Autodesk Inventor part; units mm, degrees
(part 2 of 2)
sketch "Sketch26" plane through (0, 0, 0) normal (0, -1, 0) x (1, 0, 0)
  circle A0 centre (0, 0) radius 28.575 construction
  spline S0 degree 2 poles (-30.1376, 4.8959) (-29.6848, 4.8568) (-29.0206, 4.4523) (-28.8189, 4.1472) knots 0 0 0 1 2 2 2
  spline S1 degree 2 poles (-28.8189, 4.1472) (-28.5829, 3.7797) (-28.4242, 2.9776) (-28.4778, 2.3575) knots 0 0 0 1 2 2 2
  line L0 (-28.4778, 2.3575) -> (-28.6284, 0.6152)
  line L1 (-28.6284, 0.6152) -> (-34.7017, 1.1402)
  line L2 (-34.7017, 1.1402) -> (-34.5626, 2.7496)
  spline S2 degree 2 poles (-34.5626, 2.7496) (-34.5065, 3.3992) (-34.3666, 4.0417) (-34.1787, 4.3229) knots 0 0 0 1 2 2 2
  spline S3 degree 2 poles (-34.1787, 4.3229) (-33.9779, 4.6378) (-33.386, 4.8891) (-33.0021, 4.8559) knots 0 0 0 1 2 2 2
  spline S4 degree 2 poles (-33.0021, 4.8559) (-32.5739, 4.8189) (-31.9339, 4.3074) (-31.7764, 3.8921) knots 0 0 0 1 2 2 2
  line L3 (-31.7764, 3.8921) -> (-31.7468, 3.8896)
  spline S5 degree 2 poles (-31.7468, 3.8896) (-31.5524, 4.4182) (-30.7184, 4.9461) (-30.1376, 4.8959) knots 0 0 0 1 2 2 2
  spline S6 degree 2 poles (-30.1759, 4.0513) (-30.5204, 4.0811) (-30.9804, 3.9225) (-31.1634, 3.6408) knots 0 0 0 1 2 2 2
  spline S7 degree 2 poles (-31.1634, 3.6408) (-31.2784, 3.4574) (-31.3766, 3.0097) (-31.4128, 2.5914) knots 0 0 0 1 2 2 2
  line L4 (-31.4128, 2.5914) -> (-31.4919, 1.6759)
  line L5 (-31.4919, 1.6759) -> (-29.2476, 1.4819)
  line L6 (-29.2476, 1.4819) -> (-29.1911, 2.1365)
  spline S8 degree 2 poles (-29.1911, 2.1365) (-29.1451, 2.6681) (-29.1908, 3.2868) (-29.3279, 3.5367) knots 0 0 0 1 2 2 2
  spline S9 degree 2 poles (-29.3279, 3.5367) (-29.4707, 3.7771) (-29.856, 4.0237) (-30.1759, 4.0513) knots 0 0 0 1 2 2 2
  spline S10 degree 2 poles (-32.9616, 4.0045) (-33.1782, 4.0232) (-33.5158, 3.9037) (-33.6233, 3.7493) knots 0 0 0 1 2 2 2
  spline S11 degree 2 poles (-33.6233, 3.7493) (-33.7486, 3.5618) (-33.8391, 3.0887) (-33.8761, 2.6605) knots 0 0 0 1 2 2 2
  line L7 (-33.8761, 2.6605) -> (-33.9429, 1.8878)
  line L8 (-33.9429, 1.8878) -> (-32.1662, 1.7342)
  line L9 (-32.1662, 1.7342) -> (-32.0871, 2.6496)
  spline S12 degree 2 poles (-32.0871, 2.6496) (-32.0543, 3.0286) (-32.102, 3.3947) (-32.2085, 3.5973) knots 0 0 0 1 2 2 2
  spline S13 degree 2 poles (-32.2085, 3.5973) (-32.3104, 3.7945) (-32.6762, 3.9798) (-32.9616, 4.0045) knots 0 0 0 1 2 2 2
  spline S14 degree 2 poles (-29.3792, 9.6703) (-28.2597, 9.3822) (-27.3168, 7.9918) (-27.5482, 7.0924) knots 0 0 0 1 2 2 2
  spline S15 degree 2 poles (-27.5482, 7.0924) (-27.7859, 6.169) (-29.3162, 5.4356) (-30.3974, 5.7138) knots 0 0 0 1 2 2 2
  spline S16 degree 2 poles (-30.3974, 5.7138) (-31.5073, 5.9995) (-32.4561, 7.4067) (-32.2271, 8.2965) knots 0 0 0 1 2 2 2
  spline S17 degree 2 poles (-32.2271, 8.2965) (-31.9956, 9.196) (-30.4939, 9.9572) (-29.3792, 9.6703) knots 0 0 0 1 2 2 2
  spline S18 degree 2 poles (-29.5774, 8.9001) (-30.4385, 9.1217) (-31.4371, 8.7104) (-31.586, 8.1316) knots 0 0 0 1 2 2 2
  spline S19 degree 2 poles (-31.586, 8.1316) (-31.735, 7.5527) (-31.0603, 6.7057) (-30.1992, 6.4841) knots 0 0 0 1 2 2 2
  spline S20 degree 2 poles (-30.1992, 6.4841) (-29.362, 6.2686) (-28.3383, 6.6785) (-28.1893, 7.2574) knots 0 0 0 1 2 2 2
  spline S21 degree 2 poles (-28.1893, 7.2574) (-28.0416, 7.8315) (-28.7258, 8.6809) (-29.5774, 8.9001) knots 0 0 0 1 2 2 2
  spline S22 degree 2 poles (-26.2499, 11.0765) (-26.4828, 10.494) (-27.4102, 10.104) (-28.1304, 10.392) knots 0 0 0 1 2 2 2
  line L10 (-28.1304, 10.392) -> (-30.4835, 11.3329)
  line L11 (-30.4835, 11.3329) -> (-30.676, 10.8513)
  line L12 (-30.676, 10.8513) -> (-31.2678, 11.0879)
  line L13 (-31.2678, 11.0879) -> (-31.0752, 11.5695)
  line L14 (-31.0752, 11.5695) -> (-32.2953, 12.0574)
  line L15 (-32.2953, 12.0574) -> (-32.0092, 12.773)
  line L16 (-32.0092, 12.773) -> (-30.789, 12.2851)
  line L17 (-30.789, 12.2851) -> (-30.2626, 13.6015)
  line L18 (-30.2626, 13.6015) -> (-29.6709, 13.3649)
  line L19 (-29.6709, 13.3649) -> (-30.1973, 12.0485)
  line L20 (-30.1973, 12.0485) -> (-28.1745, 11.2396)
  spline S23 degree 2 poles (-28.1745, 11.2396) (-27.8534, 11.1112) (-27.4911, 10.9929) (-27.3085, 11.0104) knots 0 0 0 1 2 2 2
  spline S24 degree 2 poles (-27.3085, 11.0104) (-27.1498, 11.0214) (-26.9012, 11.2572) (-26.8022, 11.5049) knots 0 0 0 1 2 2 2
  spline S25 degree 2 poles (-26.8022, 11.5049) (-26.7325, 11.6792) (-26.7078, 12.047) (-26.7105, 12.1332) knots 0 0 0 1 2 2 2
  line L21 (-26.7105, 12.1332) -> (-26.694, 12.1745)
  line L22 (-26.694, 12.1745) -> (-26.0518, 11.9177)
  spline S26 degree 2 poles (-26.0518, 11.9177) (-26.0775, 11.6939) (-26.1784, 11.2554) (-26.2499, 11.0765) knots 0 0 0 1 2 2 2
  spline S27 degree 2 poles (-25.0386, 13.5947) (-25.3275, 13.0378) (-26.2886, 12.7405) (-26.9771, 13.0976) knots 0 0 0 1 2 2 2
  line L23 (-26.9771, 13.0976) -> (-29.2267, 14.2645)
  line L24 (-29.2267, 14.2645) -> (-29.4655, 13.8041)
  line L25 (-29.4655, 13.8041) -> (-30.0312, 14.0975)
  line L26 (-30.0312, 14.0975) -> (-29.7924, 14.558)
  line L27 (-29.7924, 14.558) -> (-30.9588, 15.163)
  line L28 (-30.9588, 15.163) -> (-30.604, 15.8471)
  line L29 (-30.604, 15.8471) -> (-29.4375, 15.2421)
  line L30 (-29.4375, 15.2421) -> (-28.7847, 16.5006)
  line L31 (-28.7847, 16.5006) -> (-28.219, 16.2072)
  line L32 (-28.219, 16.2072) -> (-28.8718, 14.9486)
  line L33 (-28.8718, 14.9486) -> (-26.938, 13.9455)
  spline S28 degree 2 poles (-26.938, 13.9455) (-26.631, 13.7863) (-26.282, 13.633) (-26.0986, 13.6325) knots 0 0 0 1 2 2 2
  spline S29 degree 2 poles (-26.0986, 13.6325) (-25.9396, 13.628) (-25.6691, 13.8383) (-25.5463, 14.0751) knots 0 0 0 1 2 2 2
  spline S30 degree 2 poles (-25.5463, 14.0751) (-25.4598, 14.2417) (-25.3992, 14.6054) (-25.3935, 14.6914) knots 0 0 0 1 2 2 2
  line L34 (-25.3935, 14.6914) -> (-25.373, 14.7309)
  line L35 (-25.373, 14.7309) -> (-24.7591, 14.4125)
  spline S31 degree 2 poles (-24.7591, 14.4125) (-24.8066, 14.1922) (-24.9499, 13.7657) (-25.0386, 13.5947) knots 0 0 0 1 2 2 2
  spline S32 degree 2 poles (-24.1836, 19.2822) (-23.2342, 18.6228) (-22.8335, 16.9913) (-23.3633, 16.2285) knots 0 0 0 1 2 2 2
  spline S33 degree 2 poles (-23.3633, 16.2285) (-23.9072, 15.4454) (-25.597, 15.2898) (-26.514, 15.9266) knots 0 0 0 1 2 2 2
  spline S34 degree 2 poles (-26.514, 15.9266) (-27.4554, 16.5803) (-27.8557, 18.2297) (-27.3316, 18.9844) knots 0 0 0 1 2 2 2
  spline S35 degree 2 poles (-27.3316, 18.9844) (-26.8018, 19.7472) (-25.129, 19.9387) (-24.1836, 19.2822) knots 0 0 0 1 2 2 2
  spline S36 degree 2 poles (-24.6373, 18.6289) (-25.3677, 19.1361) (-26.4469, 19.0977) (-26.7878, 18.6068) knots 0 0 0 1 2 2 2
  spline S37 degree 2 poles (-26.7878, 18.6068) (-27.1288, 18.1158) (-26.7907, 17.0871) (-26.0604, 16.5799) knots 0 0 0 1 2 2 2
  spline S38 degree 2 poles (-26.0604, 16.5799) (-25.3503, 16.0867) (-24.248, 16.1151) (-23.907, 16.6061) knots 0 0 0 1 2 2 2
  spline S39 degree 2 poles (-23.907, 16.6061) (-23.5689, 17.093) (-23.9151, 18.1273) (-24.6373, 18.6289) knots 0 0 0 1 2 2 2
  line L36 (-18.1124, 22.2132) -> (-19.9399, 24.1292)
  spline S40 degree 2 poles (-19.9399, 24.1292) (-20.1582, 24.358) (-20.5656, 24.7135) (-20.725, 24.7662) knots 0 0 0 1 2 2 2
  spline S41 degree 2 poles (-20.725, 24.7662) (-20.8948, 24.8296) (-21.2219, 24.736) (-21.4114, 24.5553) knots 0 0 0 1 2 2 2
  spline S42 degree 2 poles (-21.4114, 24.5553) (-21.583, 24.3916) (-21.775, 23.8057) (-21.7914, 23.4077) knots 0 0 0 1 2 2 2
  spline S43 degree 2 poles (-21.7914, 23.4077) (-21.7401, 23.3611) (-21.5999, 23.2285) (-21.5113, 23.1356) knots 0 0 0 1 2 2 2
  line L37 (-21.5113, 23.1356) -> (-19.4314, 20.955)
  line L38 (-19.4314, 20.955) -> (-19.9891, 20.4231)
  line L39 (-19.9891, 20.4231) -> (-21.8166, 22.3391)
  spline S44 degree 2 poles (-21.8166, 22.3391) (-22.0348, 22.5679) (-22.4422, 22.9235) (-22.6017, 22.9761) knots 0 0 0 1 2 2 2
  spline S45 degree 2 poles (-22.6017, 22.9761) (-22.7714, 23.0395) (-23.0986, 22.9459) (-23.2881, 22.7652) knots 0 0 0 1 2 2 2
  spline S46 degree 2 poles (-23.2881, 22.7652) (-23.4668, 22.5948) (-23.6488, 21.9911) (-23.6676, 21.6386) knots 0 0 0 1 2 2 2
  line L40 (-23.6676, 21.6386) -> (-21.3081, 19.165)
  line L41 (-21.3081, 19.165) -> (-21.8657, 18.6331)
  line L42 (-21.8657, 18.6331) -> (-25.0231, 21.9432)
  line L43 (-25.0231, 21.9432) -> (-24.4654, 22.4751)
  line L44 (-24.4654, 22.4751) -> (-24.1177, 22.1105)
  spline S47 degree 2 poles (-24.1177, 22.1105) (-24.1076, 22.5365) (-23.9071, 23.1852) (-23.6497, 23.4307) knots 0 0 0 1 2 2 2
  spline S48 degree 2 poles (-23.6497, 23.4307) (-23.3566, 23.7103) (-22.6469, 23.8752) (-22.2391, 23.6839) knots 0 0 0 1 2 2 2
  spline S49 degree 2 poles (-22.2391, 23.6839) (-22.2547, 24.2083) (-22.0518, 24.9548) (-21.773, 25.2207) knots 0 0 0 1 2 2 2
  spline S50 degree 2 poles (-21.773, 25.2207) (-21.5585, 25.4253) (-21.0821, 25.6272) (-20.8102, 25.5998) knots 0 0 0 1 2 2 2
  spline S51 degree 2 poles (-20.8102, 25.5998) (-20.5347, 25.5758) (-19.9585, 25.2652) (-19.6346, 24.9256) knots 0 0 0 1 2 2 2
  line L45 (-19.6346, 24.9256) -> (-17.5547, 22.7451)
  line L46 (-17.5547, 22.7451) -> (-18.1124, 22.2132)
  line L47 (-10.4075, 26.7042) -> (-11.1374, 26.3526)
  line L48 (-11.1374, 26.3526) -> (-12.4323, 29.0407)
  line L49 (-12.4323, 29.0407) -> (-14.9602, 27.823)
  line L50 (-14.9602, 27.823) -> (-13.6653, 25.1348)
  line L51 (-13.6653, 25.1348) -> (-14.3952, 24.7832)
  line L52 (-14.3952, 24.7832) -> (-17.0408, 30.2752)
  line L53 (-17.0408, 30.2752) -> (-16.3109, 30.6268)
  line L54 (-16.3109, 30.6268) -> (-15.2732, 28.4727)
  line L55 (-15.2732, 28.4727) -> (-12.7453, 29.6905)
  line L56 (-12.7453, 29.6905) -> (-13.783, 31.8446)
  line L57 (-13.783, 31.8446) -> (-13.0531, 32.1962)
  line L58 (-13.0531, 32.1962) -> (-10.4075, 26.7042)
  spline S52 degree 2 poles (-7.3546, 27.507) (-8.4106, 27.2112) (-9.9031, 28.0705) (-10.2096, 29.1646) knots 0 0 0 1 2 2 2
  spline S53 degree 2 poles (-10.2096, 29.1646) (-10.5108, 30.2397) (-9.7405, 31.8303) (-8.832, 32.0849) knots 0 0 0 1 2 2 2
  spline S54 degree 2 poles (-8.832, 32.0849) (-8.4229, 32.1995) (-7.7236, 32.1389) (-7.4199, 31.952) knots 0 0 0 1 2 2 2
  spline S55 degree 2 poles (-7.4199, 31.952) (-7.1114, 31.7666) (-6.6554, 31.1094) (-6.5075, 30.5814) knots 0 0 0 1 2 2 2
  line L59 (-6.5075, 30.5814) -> (-6.3942, 30.177)
  line L60 (-6.3942, 30.177) -> (-9.4433, 29.3228)
  spline S56 degree 2 poles (-9.4433, 29.3228) (-9.2288, 28.557) (-8.2303, 27.9594) (-7.5453, 28.1513) knots 0 0 0 1 2 2 2
  spline S57 degree 2 poles (-7.5453, 28.1513) (-7.3027, 28.2193) (-6.8624, 28.4606) (-6.6961, 28.5995) knots 0 0 0 1 2 2 2
  spline S58 degree 2 poles (-6.6961, 28.5995) (-6.523, 28.7507) (-6.2937, 28.9944) (-6.2247, 29.0959) knots 0 0 0 1 2 2 2
  line L61 (-6.2247, 29.0959) -> (-6.1819, 29.1079)
  line L62 (-6.1819, 29.1079) -> (-5.9553, 28.2992)
  spline S59 degree 2 poles (-5.9553, 28.2992) (-6.0691, 28.2109) (-6.4165, 27.9494) (-6.5567, 27.8639) knots 0 0 0 1 2 2 2
  spline S60 degree 2 poles (-6.5567, 27.8639) (-6.7535, 27.7421) (-7.0882, 27.5817) (-7.3546, 27.507) knots 0 0 0 1 2 2 2
  spline S61 degree 2 poles (-7.2758, 30.5405) (-7.3693, 30.8376) (-7.6156, 31.2406) (-7.7758, 31.3547) knots 0 0 0 1 2 2 2
  spline S62 degree 2 poles (-7.7758, 31.3547) (-7.9509, 31.4852) (-8.4045, 31.5479) (-8.7042, 31.464) knots 0 0 0 1 2 2 2
  spline S63 degree 2 poles (-8.7042, 31.464) (-8.9991, 31.3814) (-9.3637, 31.0894) (-9.4869, 30.8702) knots 0 0 0 1 2 2 2
  spline S64 degree 2 poles (-9.4869, 30.8702) (-9.6041, 30.6476) (-9.6568, 30.1762) (-9.6019, 29.8889) knots 0 0 0 1 2 2 2
  line L63 (-9.6019, 29.8889) -> (-7.2758, 30.5405)
  line L64 (-1.5038, 28.6079) -> (-2.4401, 28.4915)
  line L65 (-2.4401, 28.4915) -> (-3.7551, 30.0605)
  line L66 (-3.7551, 30.0605) -> (-4.6756, 28.2138)
  line L67 (-4.6756, 28.2138) -> (-5.5433, 28.106)
  line L68 (-5.5433, 28.106) -> (-4.2493, 30.5517)
  line L69 (-4.2493, 30.5517) -> (-6.0927, 32.6473)
  line L70 (-6.0927, 32.6473) -> (-5.1563, 32.7637)
  line L71 (-5.1563, 32.7637) -> (-3.8481, 31.2088)
  line L72 (-3.8481, 31.2088) -> (-2.9356, 33.0396)
  line L73 (-2.9356, 33.0396) -> (-2.0679, 33.1475)
  line L74 (-2.0679, 33.1475) -> (-3.3533, 30.7128)
  line L75 (-3.3533, 30.7128) -> (-1.5038, 28.6079)
  line L76 (0.5107, 31.9833) -> (-0.4674, 31.9839)
  line L77 (-0.4674, 31.9839) -> (-0.4667, 33.1498)
  line L78 (-0.4667, 33.1498) -> (0.5115, 33.1491)
  line L79 (0.5115, 33.1491) -> (0.5107, 31.9833)
  line L80 (0.5084, 28.5747) -> (-0.4697, 28.5753)
  line L81 (-0.4697, 28.5753) -> (-0.469, 29.7412)
  line L82 (-0.469, 29.7412) -> (0.5092, 29.7405)
  line L83 (0.5092, 29.7405) -> (0.5084, 28.5747)
  spline S65 degree 2 poles (8.9249, 30.4001) (8.5607, 28.801) (7.2899, 27.5147) (6.3217, 27.7352) knots 0 0 0 1 2 2 2
  spline S66 degree 2 poles (6.3217, 27.7352) (5.3391, 27.959) (4.7669, 29.6954) (5.1234, 31.2609) knots 0 0 0 1 2 2 2
  spline S67 degree 2 poles (5.1234, 31.2609) (5.4898, 32.8696) (6.7584, 34.1463) (7.7313, 33.9247) knots 0 0 0 1 2 2 2
  spline S68 degree 2 poles (7.7313, 33.9247) (8.7091, 33.702) (9.2781, 31.9511) (8.9249, 30.4001) knots 0 0 0 1 2 2 2
  spline S69 degree 2 poles (7.4912, 28.8216) (7.6738, 29.0891) (7.9763, 29.9727) (8.1157, 30.5844) knots 0 0 0 1 2 2 2
  spline S70 degree 2 poles (8.1157, 30.5844) (8.255, 31.1962) (8.3638, 32.1188) (8.3125, 32.4497) knots 0 0 0 1 2 2 2
  spline S71 degree 2 poles (8.3125, 32.4497) (8.2612, 32.7806) (7.9134, 33.1891) (7.5811, 33.2648) knots 0 0 0 1 2 2 2
  spline S72 degree 2 poles (7.5811, 33.2648) (7.2487, 33.3405) (6.7487, 33.125) (6.5522, 32.8405) knots 0 0 0 1 2 2 2
  spline S73 degree 2 poles (6.5522, 32.8405) (6.3627, 32.5644) (6.0653, 31.6594) (5.9326, 31.0766) knots 0 0 0 1 2 2 2
  spline S74 degree 2 poles (5.9326, 31.0766) (5.79, 30.4504) (5.6762, 29.5947) (5.7268, 29.2387) knots 0 0 0 1 2 2 2
  spline S75 degree 2 poles (5.7268, 29.2387) (5.7722, 28.9041) (6.1252, 28.4741) (6.472, 28.3951) knots 0 0 0 1 2 2 2
  spline S76 degree 2 poles (6.472, 28.3951) (6.7995, 28.3205) (7.2995, 28.536) (7.4912, 28.8216) knots 0 0 0 1 2 2 2
  line L84 (10.2051, 26.695) -> (9.2857, 27.0287)
  line L85 (9.2857, 27.0287) -> (9.6835, 28.1246)
  line L86 (9.6835, 28.1246) -> (10.6029, 27.7908)
  line L87 (10.6029, 27.7908) -> (10.2051, 26.695)
  spline S77 degree 2 poles (15.5351, 26.3257) (15.335, 25.9342) (14.7426, 25.3937) (14.3879, 25.2643) knots 0 0 0 1 2 2 2
  spline S78 degree 2 poles (14.3879, 25.2643) (14.0333, 25.1349) (13.2053, 25.1974) (12.7831, 25.4133) knots 0 0 0 1 2 2 2
  spline S79 degree 2 poles (12.7831, 25.4133) (12.396, 25.6111) (11.727, 26.1693) (11.5196, 26.4473) knots 0 0 0 1 2 2 2
  line L88 (11.5196, 26.4473) -> (11.913, 27.2171)
  line L89 (11.913, 27.2171) -> (11.9658, 27.1901)
  spline S80 degree 2 poles (11.9658, 27.1901) (12.0179, 27.0858) (12.2493, 26.7679) (12.4025, 26.6008) knots 0 0 0 1 2 2 2
  spline S81 degree 2 poles (12.4025, 26.6008) (12.5798, 26.4159) (12.8934, 26.1502) (13.1177, 26.0355) knots 0 0 0 1 2 2 2
  spline S82 degree 2 poles (13.1177, 26.0355) (13.3377, 25.9231) (13.8321, 25.8702) (14.0693, 25.9653) knots 0 0 0 1 2 2 2
  spline S83 degree 2 poles (14.0693, 25.9653) (14.2889, 26.0583) (14.65, 26.4175) (14.7984, 26.7078) knots 0 0 0 1 2 2 2
  spline S84 degree 2 poles (14.7984, 26.7078) (14.9467, 26.9981) (14.9772, 27.4486) (14.8906, 27.6482) knots 0 0 0 1 2 2 2
  spline S85 degree 2 poles (14.8906, 27.6482) (14.8063, 27.8632) (14.4073, 28.2114) (14.1302, 28.353) knots 0 0 0 1 2 2 2
  spline S86 degree 2 poles (14.1302, 28.353) (13.8311, 28.5059) (13.19, 28.717) (12.9894, 28.7696) knots 0 0 0 1 2 2 2
  line L90 (12.9894, 28.7696) -> (14.4193, 31.5673)
  line L91 (14.4193, 31.5673) -> (17.3973, 30.0453)
  line L92 (17.3973, 30.0453) -> (17.0713, 29.4074)
  line L93 (17.0713, 29.4074) -> (14.7927, 30.572)
  line L94 (14.7927, 30.572) -> (14.0531, 29.1248)
  spline S87 degree 2 poles (14.0531, 29.1248) (14.194, 29.0749) (14.4559, 28.9577) (14.5615, 28.9038) knots 0 0 0 1 2 2 2
  spline S88 degree 2 poles (14.5615, 28.9038) (14.9793, 28.6902) (15.4859, 28.2593) (15.6464, 27.9221) knots 0 0 0 1 2 2 2
  spline S89 degree 2 poles (15.6464, 27.9221) (15.8113, 27.5826) (15.7869, 26.8184) (15.5351, 26.3257) knots 0 0 0 1 2 2 2
  line L95 (18.4323, 21.9193) -> (15.3996, 24.1408)
  line L96 (15.3996, 24.1408) -> (15.9105, 24.8382)
  spline S90 degree 2 poles (15.9105, 24.8382) (16.462, 24.9057) (17.4613, 25.0494) (17.9651, 25.1519) knots 0 0 0 1 2 2 2
  spline S91 degree 2 poles (17.9651, 25.1519) (18.9795, 25.358) (19.9329, 25.7985) (20.2219, 26.1931) knots 0 0 0 1 2 2 2
  spline S92 degree 2 poles (20.2219, 26.1931) (20.3737, 26.4003) (20.4739, 26.8046) (20.4313, 26.9889) knots 0 0 0 1 2 2 2
  spline S93 degree 2 poles (20.4313, 26.9889) (20.3887, 27.1731) (20.1588, 27.4946) (19.9755, 27.6289) knots 0 0 0 1 2 2 2
  spline S94 degree 2 poles (19.9755, 27.6289) (19.8002, 27.7574) (19.3773, 27.9324) (19.1643, 27.9844) knots 0 0 0 1 2 2 2
  spline S95 degree 2 poles (19.1643, 27.9844) (18.9839, 28.0308) (18.6081, 28.0611) (18.4875, 28.0637) knots 0 0 0 1 2 2 2
  line L97 (18.4875, 28.0637) -> (18.4517, 28.09)
  line L98 (18.4517, 28.09) -> (18.9654, 28.7914)
  spline S96 degree 2 poles (18.9654, 28.7914) (19.2417, 28.7421) (20.114, 28.4032) (20.4408, 28.1638) knots 0 0 0 1 2 2 2
  spline S97 degree 2 poles (20.4408, 28.1638) (21.1302, 27.6587) (21.3731, 26.3602) (20.9177, 25.7385) knots 0 0 0 1 2 2 2
  spline S98 degree 2 poles (20.9177, 25.7385) (20.7046, 25.4476) (20.213, 25.0606) (19.9416, 24.941) knots 0 0 0 1 2 2 2
  spline S99 degree 2 poles (19.9416, 24.941) (19.6644, 24.8134) (19.0083, 24.6449) (18.6681, 24.5818) knots 0 0 0 1 2 2 2
  spline S100 degree 2 poles (18.6681, 24.5818) (18.1091, 24.4708) (16.8166, 24.303) (16.4348, 24.2582) knots 0 0 0 1 2 2 2
  line L99 (16.4348, 24.2582) -> (18.8498, 22.4891)
  line L100 (18.8498, 22.4891) -> (18.4323, 21.9193)
  line L101 (21.6843, 18.7082) -> (19.0435, 21.3839)
  line L102 (19.0435, 21.3839) -> (19.6588, 21.9911)
  spline S101 degree 2 poles (19.6588, 21.9911) (20.2141, 21.97) (21.2235, 21.9529) (21.7372, 21.974) knots 0 0 0 1 2 2 2
  spline S102 degree 2 poles (21.7372, 21.974) (22.7714, 22.0161) (23.7828, 22.2994) (24.1309, 22.6429) knots 0 0 0 1 2 2 2
  spline S103 degree 2 poles (24.1309, 22.6429) (24.3138, 22.8234) (24.477, 23.2066) (24.4642, 23.3953) knots 0 0 0 1 2 2 2
  spline S104 degree 2 poles (24.4642, 23.3953) (24.4515, 23.584) (24.2757, 23.938) (24.116, 24.0997) knots 0 0 0 1 2 2 2
  spline S105 degree 2 poles (24.116, 24.0997) (23.9634, 24.2544) (23.5737, 24.4945) (23.3717, 24.5797) knots 0 0 0 1 2 2 2
  spline S106 degree 2 poles (23.3717, 24.5797) (23.201, 24.6541) (22.8348, 24.7439) (22.7162, 24.7656) knots 0 0 0 1 2 2 2
  line L103 (22.7162, 24.7656) -> (22.6849, 24.7973)
  line L104 (22.6849, 24.7973) -> (23.3037, 25.408)
  spline S107 degree 2 poles (23.3037, 25.408) (23.5686, 25.3154) (24.3759, 24.842) (24.6605, 24.5537) knots 0 0 0 1 2 2 2
  spline S108 degree 2 poles (24.6605, 24.5537) (25.2608, 23.9455) (25.294, 22.6248) (24.7455, 22.0835) knots 0 0 0 1 2 2 2
  spline S109 degree 2 poles (24.7455, 22.0835) (24.4889, 21.8302) (23.9419, 21.5263) (23.655, 21.4514) knots 0 0 0 1 2 2 2
  spline S110 degree 2 poles (23.655, 21.4514) (23.361, 21.3695) (22.6864, 21.3075) (22.3406, 21.2993) knots 0 0 0 1 2 2 2
  spline S111 degree 2 poles (22.3406, 21.2993) (21.771, 21.2786) (20.4683, 21.3186) (20.0842, 21.3351) knots 0 0 0 1 2 2 2
  line L105 (20.0842, 21.3351) -> (22.1871, 19.2044)
  line L106 (22.1871, 19.2044) -> (21.6843, 18.7082)
  spline S112 degree 2 poles (25.9239, 16.1968) (25.5658, 15.9416) (24.7909, 15.7352) (24.4165, 15.7839) knots 0 0 0 1 2 2 2
  spline S113 degree 2 poles (24.4165, 15.7839) (24.0422, 15.8326) (23.3363, 16.2698) (23.0611, 16.6561) knots 0 0 0 1 2 2 2
  spline S114 degree 2 poles (23.0611, 16.6561) (22.8089, 17.0101) (22.4727, 17.8139) (22.4168, 18.1562) knots 0 0 0 1 2 2 2
  line L107 (22.4168, 18.1562) -> (23.1209, 18.6579)
  line L108 (23.1209, 18.6579) -> (23.1553, 18.6096)
  spline S115 degree 2 poles (23.1553, 18.6096) (23.1534, 18.493) (23.2121, 18.1042) (23.271, 17.8853) knots 0 0 0 1 2 2 2
  spline S116 degree 2 poles (23.271, 17.8853) (23.3431, 17.6395) (23.4989, 17.2591) (23.645, 17.0539) knots 0 0 0 1 2 2 2
  spline S117 degree 2 poles (23.645, 17.0539) (23.7884, 16.8528) (24.2027, 16.5778) (24.4571, 16.5528) knots 0 0 0 1 2 2 2
  spline S118 degree 2 poles (24.4571, 16.5528) (24.6948, 16.5341) (25.1808, 16.6863) (25.4463, 16.8755) knots 0 0 0 1 2 2 2
  spline S119 degree 2 poles (25.4463, 16.8755) (25.7119, 17.0647) (25.9466, 17.4504) (25.9618, 17.6674) knots 0 0 0 1 2 2 2
  spline S120 degree 2 poles (25.9618, 17.6674) (25.9862, 17.8971) (25.7926, 18.39) (25.612, 18.6435) knots 0 0 0 1 2 2 2
  spline S121 degree 2 poles (25.612, 18.6435) (25.4171, 18.9171) (24.9456, 19.4) (24.7919, 19.5392) knots 0 0 0 1 2 2 2
  line L109 (24.7919, 19.5392) -> (27.3507, 21.3623)
  line L110 (27.3507, 21.3623) -> (29.2914, 18.6386)
  line L111 (29.2914, 18.6386) -> (28.708, 18.223)
  line L112 (28.708, 18.223) -> (27.2231, 20.307)
  line L113 (27.2231, 20.307) -> (25.8994, 19.3639)
  spline S122 degree 2 poles (25.8994, 19.3639) (26.0015, 19.2546) (26.1799, 19.0299) (26.2487, 18.9333) knots 0 0 0 1 2 2 2
  spline S123 degree 2 poles (26.2487, 18.9333) (26.521, 18.5511) (26.7718, 17.9352) (26.7587, 17.562) knots 0 0 0 1 2 2 2
  spline S124 degree 2 poles (26.7587, 17.562) (26.7485, 17.1847) (26.3745, 16.5178) (25.9239, 16.1968) knots 0 0 0 1 2 2 2
  line L114 (26.8479, 9.8544) -> (25.9436, 12.0357)
  line L115 (25.9436, 12.0357) -> (26.5186, 12.2741)
  line L116 (26.5186, 12.2741) -> (26.8156, 11.5576)
  line L117 (26.8156, 11.5576) -> (31.297, 13.4153)
  line L118 (31.297, 13.4153) -> (30.9999, 14.1318)
  line L119 (30.9999, 14.1318) -> (31.5749, 14.3701)
  line L120 (31.5749, 14.3701) -> (32.4792, 12.1888)
  line L121 (32.4792, 12.1888) -> (31.9042, 11.9505)
  line L122 (31.9042, 11.9505) -> (31.6072, 12.6669)
  line L123 (31.6072, 12.6669) -> (27.1259, 10.8092)
  line L124 (27.1259, 10.8092) -> (27.4229, 10.0927)
  line L125 (27.4229, 10.0927) -> (26.8479, 9.8544)
  spline S125 degree 2 poles (31.3296, 4.9821) (30.5185, 4.7844) (29.0527, 5.1236) (28.5534, 5.5866) knots 0 0 0 1 2 2 2
  spline S126 degree 2 poles (28.5534, 5.5866) (28.1602, 5.9687) (27.7424, 6.8482) (27.5669, 7.5681) knots 0 0 0 1 2 2 2
  line L126 (27.5669, 7.5681) -> (27.2345, 8.9311)
  line L127 (27.2345, 8.9311) -> (33.157, 10.3752)
  line L128 (33.157, 10.3752) -> (33.4858, 9.0265)
  spline S127 degree 2 poles (33.4858, 9.0265) (33.6895, 8.1914) (33.6716, 7.1803) (33.5327, 6.7905) knots 0 0 0 1 2 2 2
  spline S128 degree 2 poles (33.5327, 6.7905) (33.2928, 6.1269) (32.1935, 5.1928) (31.3296, 4.9821) knots 0 0 0 1 2 2 2
  spline S129 degree 2 poles (31.1391, 5.8052) (31.8206, 5.9713) (32.6753, 6.6577) (32.84, 7.1708) knots 0 0 0 1 2 2 2
  spline S130 degree 2 poles (32.84, 7.1708) (32.95, 7.5332) (32.9436, 8.2892) (32.8137, 8.822) knots 0 0 0 1 2 2 2
  line L129 (32.8137, 8.822) -> (32.6674, 9.4219)
  line L130 (32.6674, 9.4219) -> (28.1079, 8.3102)
  line L131 (28.1079, 8.3102) -> (28.2542, 7.7103)
  spline S131 degree 2 poles (28.2542, 7.7103) (28.3818, 7.1871) (28.7428, 6.4362) (29.0468, 6.1696) knots 0 0 0 1 2 2 2
  spline S132 degree 2 poles (29.0468, 6.1696) (29.4258, 5.8247) (30.448, 5.6367) (31.1391, 5.8052) knots 0 0 0 1 2 2 2
  line L132 (28.5071, 2.0292) -> (28.4209, 3.0035)
  line L133 (28.4209, 3.0035) -> (29.5822, 3.1062)
  line L134 (29.5822, 3.1062) -> (29.6684, 2.1318)
  line L135 (29.6684, 2.1318) -> (28.5071, 2.0292)
  line L136 (31.9024, 2.3293) -> (31.8163, 3.3037)
  line L137 (31.8163, 3.3037) -> (32.9776, 3.4063)
  line L138 (32.9776, 3.4063) -> (33.0638, 2.432)
  line L139 (33.0638, 2.432) -> (31.9024, 2.3293)
  line L140 (28.0978, -5.4439) -> (28.4983, -2.4971)
  line L141 (28.4983, -2.4971) -> (29.1151, -2.5809)
  line L142 (29.1151, -2.5809) -> (28.9661, -3.6774)
  line L143 (28.9661, -3.6774) -> (33.0143, -4.2276)
  line L144 (33.0143, -4.2276) -> (33.1633, -3.1311)
  line L145 (33.1633, -3.1311) -> (33.7164, -3.2063)
  spline S133 degree 2 poles (33.7164, -3.2063) (33.6319, -3.8279) (33.9045, -4.4632) (34.3887, -4.5689) knots 0 0 0 1 2 2 2
  line L146 (34.3887, -4.5689) -> (34.3036, -5.1955)
  line L147 (34.3036, -5.1955) -> (28.8603, -4.4557)
  line L148 (28.8603, -4.4557) -> (28.7146, -5.5277)
  line L149 (28.7146, -5.5277) -> (28.0978, -5.4439)
  line L150 (27.4952, -7.7961) -> (27.746, -6.8507)
  line L151 (27.746, -6.8507) -> (28.8729, -7.1497)
  line L152 (28.8729, -7.1497) -> (28.6221, -8.0951)
  line L153 (28.6221, -8.0951) -> (27.4952, -7.7961)
  spline S134 degree 2 poles (27.6004, -13.1378) (27.1927, -12.9733) (26.6017, -12.4311) (26.4414, -12.0894) knots 0 0 0 1 2 2 2
  spline S135 degree 2 poles (26.4414, -12.0894) (26.281, -11.7476) (26.2698, -10.9174) (26.4473, -10.4776) knots 0 0 0 1 2 2 2
  spline S136 degree 2 poles (26.4473, -10.4776) (26.61, -10.0745) (27.1067, -9.3587) (27.3652, -9.1274) knots 0 0 0 1 2 2 2
  line L154 (27.3652, -9.1274) -> (28.1669, -9.451)
  line L155 (28.1669, -9.451) -> (28.1447, -9.5059)
  spline S137 degree 2 poles (28.1447, -9.5059) (28.0454, -9.5671) (27.7492, -9.8258) (27.5964, -9.9932) knots 0 0 0 1 2 2 2
  spline S138 degree 2 poles (27.5964, -9.9932) (27.4279, -10.1862) (27.1911, -10.5221) (27.0968, -10.7558) knots 0 0 0 1 2 2 2
  spline S139 degree 2 poles (27.0968, -10.7558) (27.0044, -10.9848) (26.9955, -11.482) (27.1113, -11.7098) knots 0 0 0 1 2 2 2
  spline S140 degree 2 poles (27.1113, -11.7098) (27.2235, -11.9203) (27.6132, -12.2481) (27.9156, -12.3701) knots 0 0 0 1 2 2 2
  spline S141 degree 2 poles (27.9156, -12.3701) (28.2179, -12.4921) (28.6693, -12.4825) (28.8604, -12.3785) knots 0 0 0 1 2 2 2
  spline S142 degree 2 poles (28.8604, -12.3785) (29.0671, -12.2755) (29.3785, -11.8472) (29.495, -11.5586) knots 0 0 0 1 2 2 2
  spline S143 degree 2 poles (29.495, -11.5586) (29.6208, -11.2471) (29.7742, -10.5898) (29.8087, -10.3854) knots 0 0 0 1 2 2 2
  line L156 (29.8087, -10.3854) -> (32.7222, -11.5613)
  line L157 (32.7222, -11.5613) -> (31.4705, -14.6626)
  line L158 (31.4705, -14.6626) -> (30.8062, -14.3945)
  line L159 (30.8062, -14.3945) -> (31.764, -12.0216)
  line L160 (31.764, -12.0216) -> (30.2569, -11.4133)
  spline S144 degree 2 poles (30.2569, -11.4133) (30.2197, -11.5581) (30.1262, -11.8293) (30.0819, -11.9393) knots 0 0 0 1 2 2 2
  spline S145 degree 2 poles (30.0819, -11.9393) (29.9062, -12.3745) (29.522, -12.9173) (29.2003, -13.1071) knots 0 0 0 1 2 2 2
  spline S146 degree 2 poles (29.2003, -13.1071) (28.8768, -13.3014) (28.1134, -13.3449) (27.6004, -13.1378) knots 0 0 0 1 2 2 2
  line L161 (29.6765, -18.4873) -> (27.7102, -17.1502)
  line L162 (27.7102, -17.1502) -> (27.9788, -16.6835)
  line L163 (27.9788, -16.6835) -> (30.1226, -17.7123)
  line L164 (30.1226, -17.7123) -> (29.6765, -18.4873)
  line L165 (30.4454, -17.1515) -> (28.4791, -15.8144)
  line L166 (28.4791, -15.8144) -> (28.7477, -15.3477)
  line L167 (28.7477, -15.3477) -> (30.8915, -16.3765)
  line L168 (30.8915, -16.3765) -> (30.4454, -17.1515)
  spline S147 degree 2 poles (22.8704, -25.2005) (22.3391, -25.1635) (21.223, -24.608) (20.6801, -24.0751) knots 0 0 0 1 2 2 2
  spline S148 degree 2 poles (20.6801, -24.0751) (20.1513, -23.556) (19.5576, -22.4472) (19.5177, -21.9096) knots 0 0 0 1 2 2 2
  spline S149 degree 2 poles (19.5177, -21.9096) (19.4775, -21.344) (19.8839, -20.3517) (20.3027, -19.9251) knots 0 0 0 1 2 2 2
  spline S150 degree 2 poles (20.3027, -19.9251) (20.7352, -19.4844) (21.727, -19.0734) (22.2722, -19.1033) knots 0 0 0 1 2 2 2
  spline S151 degree 2 poles (22.2722, -19.1033) (22.807, -19.1368) (23.9196, -19.7028) (24.4555, -20.2288) knots 0 0 0 1 2 2 2
  spline S152 degree 2 poles (24.4555, -20.2288) (25.0019, -20.7652) (25.5675, -21.8533) (25.6215, -22.3978) knots 0 0 0 1 2 2 2
  spline S153 degree 2 poles (25.6215, -22.3978) (25.6614, -22.9354) (25.2655, -23.9381) (24.8364, -24.3753) knots 0 0 0 1 2 2 2
  spline S154 degree 2 poles (24.8364, -24.3753) (24.4004, -24.8195) (23.3911, -25.2271) (22.8704, -25.2005) knots 0 0 0 1 2 2 2
  spline S155 degree 2 poles (21.2718, -23.4722) (21.702, -23.8944) (22.5517, -24.3616) (22.9364, -24.4069) knots 0 0 0 1 2 2 2
  spline S156 degree 2 poles (22.9364, -24.4069) (23.3315, -24.4556) (24.0347, -24.1906) (24.3323, -23.8874) knots 0 0 0 1 2 2 2
  spline S157 degree 2 poles (24.3323, -23.8874) (24.6403, -23.5736) (24.8854, -22.8867) (24.8292, -22.4785) knots 0 0 0 1 2 2 2
  spline S158 degree 2 poles (24.8292, -22.4785) (24.7767, -22.0877) (24.2868, -21.2469) (23.8638, -20.8317) knots 0 0 0 1 2 2 2
  spline S159 degree 2 poles (23.8638, -20.8317) (23.0071, -19.9908) (21.3916, -19.8171) (20.7998, -20.42) knots 0 0 0 1 2 2 2
  spline S160 degree 2 poles (20.7998, -20.42) (20.2081, -21.0228) (20.4152, -22.6313) (21.2718, -23.4722) knots 0 0 0 1 2 2 2
  spline S161 degree 2 poles (15.5041, -27.6765) (15.0381, -26.9837) (14.8498, -25.4911) (15.1117, -24.8625) knots 0 0 0 1 2 2 2
  spline S162 degree 2 poles (15.1117, -24.8625) (15.3343, -24.3615) (16.0152, -23.6654) (16.6301, -23.2518) knots 0 0 0 1 2 2 2
  line L169 (16.6301, -23.2518) -> (17.7942, -22.4689)
  line L170 (17.7942, -22.4689) -> (21.1964, -27.5272)
  line L171 (21.1964, -27.5272) -> (20.0445, -28.3019)
  spline S163 degree 2 poles (20.0445, -28.3019) (19.3313, -28.7816) (18.3763, -29.1143) (17.9625, -29.1188) knots 0 0 0 1 2 2 2
  spline S164 degree 2 poles (17.9625, -29.1188) (17.2569, -29.123) (16.0003, -28.4143) (15.5041, -27.6765) knots 0 0 0 1 2 2 2
  spline S165 degree 2 poles (16.2105, -27.2132) (16.602, -27.7953) (17.5415, -28.3601) (18.0799, -28.3373) knots 0 0 0 1 2 2 2
  spline S166 degree 2 poles (18.0799, -28.3373) (18.4579, -28.3152) (19.1652, -28.0479) (19.6202, -27.7419) knots 0 0 0 1 2 2 2
  line L172 (19.6202, -27.7419) -> (20.1326, -27.3973)
  line L173 (20.1326, -27.3973) -> (17.5134, -23.5031)
  line L174 (17.5134, -23.5031) -> (17.0011, -23.8477)
  spline S167 degree 2 poles (17.0011, -23.8477) (16.5543, -24.1482) (15.9744, -24.7466) (15.8293, -25.124) knots 0 0 0 1 2 2 2
  spline S168 degree 2 poles (15.8293, -25.124) (15.6367, -25.5988) (15.8135, -26.623) (16.2105, -27.2132) knots 0 0 0 1 2 2 2
  line L175 (13.2128, -29.131) -> (14.0973, -28.7134)
  line L176 (14.0973, -28.7134) -> (14.595, -29.7676)
  line L177 (14.595, -29.7676) -> (13.7105, -30.1852)
  line L178 (13.7105, -30.1852) -> (13.2128, -29.131)
  line L179 (11.7575, -26.0486) -> (12.642, -25.631)
  line L180 (12.642, -25.631) -> (13.1398, -26.6853)
  line L181 (13.1398, -26.6853) -> (12.2553, -27.1029)
  line L182 (12.2553, -27.1029) -> (11.7575, -26.0486)
  spline S169 degree 2 poles (7.5616, -33.2445) (7.7786, -33.1964) (8.1844, -32.9953) (8.3736, -32.8674) knots 0 0 0 1 2 2 2
  spline S170 degree 2 poles (8.3736, -32.8674) (8.5484, -32.7427) (8.7945, -32.5061) (8.8884, -32.4043) knots 0 0 0 1 2 2 2
  line L183 (8.8884, -32.4043) -> (8.9366, -32.3937)
  line L184 (8.9366, -32.3937) -> (9.1235, -33.2377)
  spline S171 degree 2 poles (9.1235, -33.2377) (8.894, -33.4353) (8.0519, -33.8595) (7.6515, -33.9481) knots 0 0 0 1 2 2 2
  spline S172 degree 2 poles (7.6515, -33.9481) (7.2464, -34.0378) (6.6072, -34.0073) (6.3227, -33.8881) knots 0 0 0 1 2 2 2
  spline S173 degree 2 poles (6.3227, -33.8881) (6.0206, -33.7576) (5.6299, -33.2724) (5.5487, -32.9058) knots 0 0 0 1 2 2 2
  spline S174 degree 2 poles (5.5487, -32.9058) (5.4398, -32.4138) (5.9217, -31.528) (6.3538, -31.3311) knots 0 0 0 1 2 2 2
  line L185 (6.3538, -31.3311) -> (6.341, -31.2733)
  spline S175 degree 2 poles (6.341, -31.2733) (6.1443, -31.2763) (5.6766, -31.1977) (5.4549, -31.0646) knots 0 0 0 1 2 2 2
  spline S176 degree 2 poles (5.4549, -31.0646) (5.2342, -30.9364) (4.8831, -30.4474) (4.7966, -30.0568) knots 0 0 0 1 2 2 2
  spline S177 degree 2 poles (4.7966, -30.0568) (4.708, -29.6564) (4.8324, -28.9155) (5.0256, -28.5995) knots 0 0 0 1 2 2 2
  spline S178 degree 2 poles (5.0256, -28.5995) (5.2262, -28.2718) (5.9023, -27.8286) (6.3701, -27.7251) knots 0 0 0 1 2 2 2
  spline S179 degree 2 poles (6.3701, -27.7251) (6.8187, -27.6258) (7.7446, -27.6485) (8.0767, -27.7318) knots 0 0 0 1 2 2 2
  line L186 (8.0767, -27.7318) -> (8.2635, -28.5759)
  line L187 (8.2635, -28.5759) -> (8.2057, -28.5887)
  spline S180 degree 2 poles (8.2057, -28.5887) (7.9143, -28.461) (6.9906, -28.3112) (6.571, -28.4041) knots 0 0 0 1 2 2 2
  spline S181 degree 2 poles (6.571, -28.4041) (6.325, -28.4586) (5.8672, -28.7218) (5.7427, -28.9366) knots 0 0 0 1 2 2 2
  spline S182 degree 2 poles (5.7427, -28.9366) (5.6231, -29.1503) (5.5482, -29.6121) (5.6198, -29.9353) knots 0 0 0 1 2 2 2
  spline S183 degree 2 poles (5.6198, -29.9353) (5.6913, -30.2584) (5.9723, -30.6364) (6.1678, -30.7196) knots 0 0 0 1 2 2 2
  spline S184 degree 2 poles (6.1678, -30.7196) (6.3633, -30.8028) (6.8418, -30.793) (7.1119, -30.7333) knots 0 0 0 1 2 2 2
  line L188 (7.1119, -30.7333) -> (7.4495, -30.6585)
  line L189 (7.4495, -30.6585) -> (7.5958, -31.3193)
  line L190 (7.5958, -31.3193) -> (7.3305, -31.378)
  spline S185 degree 2 poles (7.3305, -31.378) (6.7951, -31.4965) (6.2331, -32.1573) (6.3409, -32.6444) knots 0 0 0 1 2 2 2
  spline S186 degree 2 poles (6.3409, -32.6444) (6.3911, -32.8711) (6.6363, -33.1559) (6.7975, -33.2214) knots 0 0 0 1 2 2 2
  spline S187 degree 2 poles (6.7975, -33.2214) (6.9694, -33.2895) (7.3542, -33.2904) (7.5616, -33.2445) knots 0 0 0 1 2 2 2
  line L191 (2.1881, -28.4952) -> (3.1619, -28.4038)
  line L192 (3.1619, -28.4038) -> (3.2709, -29.5646)
  line L193 (3.2709, -29.5646) -> (2.297, -29.656)
  line L194 (2.297, -29.656) -> (2.1881, -28.4952)
  line L195 (-2.7928, -28.5027) -> (0.9648, -28.6181)
  line L196 (0.9648, -28.6181) -> (0.9382, -29.4822)
  spline S188 degree 2 poles (0.9382, -29.4822) (0.5217, -29.85) (-0.2209, -30.5339) (-0.5782, -30.9035) knots 0 0 0 1 2 2 2
  spline S189 degree 2 poles (-0.5782, -30.9035) (-1.2979, -31.6475) (-1.8347, -32.5503) (-1.8497, -33.0391) knots 0 0 0 1 2 2 2
  spline S190 degree 2 poles (-1.8497, -33.0391) (-1.8576, -33.2959) (-1.7114, -33.6859) (-1.572, -33.8137) knots 0 0 0 1 2 2 2
  spline S191 degree 2 poles (-1.572, -33.8137) (-1.4326, -33.9415) (-1.0612, -34.0765) (-0.834, -34.0835) knots 0 0 0 1 2 2 2
  spline S192 degree 2 poles (-0.834, -34.0835) (-0.6168, -34.0901) (-0.169, -33.9952) (0.036, -33.9174) knots 0 0 0 1 2 2 2
  spline S193 degree 2 poles (0.036, -33.9174) (0.2109, -33.8536) (0.538, -33.666) (0.6388, -33.5999) knots 0 0 0 1 2 2 2
  line L197 (0.6388, -33.5999) -> (0.6833, -33.6012)
  line L198 (0.6833, -33.6012) -> (0.6566, -34.4703)
  spline S194 degree 2 poles (0.6566, -34.4703) (0.401, -34.586) (-0.5101, -34.8002) (-0.915, -34.7877) knots 0 0 0 1 2 2 2
  spline S195 degree 2 poles (-0.915, -34.7877) (-1.7692, -34.7615) (-2.7043, -33.8284) (-2.6806, -33.0581) knots 0 0 0 1 2 2 2
  spline S196 degree 2 poles (-2.6806, -33.0581) (-2.6696, -32.6976) (-2.4832, -32.1004) (-2.3272, -31.8482) knots 0 0 0 1 2 2 2
  spline S197 degree 2 poles (-2.3272, -31.8482) (-2.1708, -31.5861) (-1.7252, -31.0759) (-1.4805, -30.8313) knots 0 0 0 1 2 2 2
  spline S198 degree 2 poles (-1.4805, -30.8313) (-1.0824, -30.4234) (-0.1117, -29.5537) (0.1778, -29.3007) knots 0 0 0 1 2 2 2
  line L199 (0.1778, -29.3007) -> (-2.8145, -29.2088)
  line L200 (-2.8145, -29.2088) -> (-2.7928, -28.5027)
  spline S199 degree 2 poles (-7.5946, -29.6092) (-7.5114, -29.1775) (-7.0928, -28.4935) (-6.7882, -28.2705) knots 0 0 0 1 2 2 2
  spline S200 degree 2 poles (-6.7882, -28.2705) (-6.4836, -28.0475) (-5.6709, -27.8771) (-5.2052, -27.9669) knots 0 0 0 1 2 2 2
  spline S201 degree 2 poles (-5.2052, -27.9669) (-4.7784, -28.0492) (-3.9805, -28.3992) (-3.7039, -28.6085) knots 0 0 0 1 2 2 2
  line L201 (-3.7039, -28.6085) -> (-3.8676, -29.4573)
  line L202 (-3.8676, -29.4573) -> (-3.9258, -29.4461)
  spline S202 degree 2 poles (-3.9258, -29.4461) (-4.0048, -29.3604) (-4.3156, -29.1194) (-4.5092, -29.0016) knots 0 0 0 1 2 2 2
  spline S203 degree 2 poles (-4.5092, -29.0016) (-4.731, -28.8733) (-5.1061, -28.7054) (-5.3535, -28.6577) knots 0 0 0 1 2 2 2
  spline S204 degree 2 poles (-5.3535, -28.6577) (-5.596, -28.611) (-6.0857, -28.6977) (-6.2871, -28.8551) knots 0 0 0 1 2 2 2
  spline S205 degree 2 poles (-6.2871, -28.8551) (-6.472, -29.0056) (-6.7189, -29.451) (-6.7806, -29.7712) knots 0 0 0 1 2 2 2
  spline S206 degree 2 poles (-6.7806, -29.7712) (-6.8423, -30.0913) (-6.7463, -30.5324) (-6.6075, -30.7) knots 0 0 0 1 2 2 2
  spline S207 degree 2 poles (-6.6075, -30.7) (-6.4667, -30.8831) (-5.9866, -31.1065) (-5.681, -31.1654) knots 0 0 0 1 2 2 2
  spline S208 degree 2 poles (-5.681, -31.1654) (-5.3511, -31.229) (-4.6766, -31.2534) (-4.4694, -31.2481) knots 0 0 0 1 2 2 2
  line L203 (-4.4694, -31.2481) -> (-5.0641, -34.3331)
  line L204 (-5.0641, -34.3331) -> (-8.348, -33.7001)
  line L205 (-8.348, -33.7001) -> (-8.2124, -32.9967)
  line L206 (-8.2124, -32.9967) -> (-5.6998, -33.4811)
  line L207 (-5.6998, -33.4811) -> (-5.3921, -31.8852)
  spline S209 degree 2 poles (-5.3921, -31.8852) (-5.5414, -31.8766) (-5.8255, -31.8369) (-5.9419, -31.8144) knots 0 0 0 1 2 2 2
  spline S210 degree 2 poles (-5.9419, -31.8144) (-6.4027, -31.7256) (-7.0092, -31.4527) (-7.2572, -31.1735) knots 0 0 0 1 2 2 2
  spline S211 degree 2 poles (-7.2572, -31.1735) (-7.5101, -30.8933) (-7.6993, -30.1525) (-7.5946, -29.6092) knots 0 0 0 1 2 2 2
  line L208 (-12.4459, -32.6737) -> (-11.5113, -30.4873)
  line L209 (-11.5113, -30.4873) -> (-11.0017, -30.6613)
  line L210 (-11.0017, -30.6613) -> (-11.5998, -32.9627)
  line L211 (-11.5998, -32.9627) -> (-12.4459, -32.6737)
  line L212 (-10.9874, -33.1719) -> (-10.0527, -30.9854)
  line L213 (-10.0527, -30.9854) -> (-9.5431, -31.1595)
  line L214 (-9.5431, -31.1595) -> (-10.1412, -33.4609)
  line L215 (-10.1412, -33.4609) -> (-10.9874, -33.1719)
  line L216 (-17.4703, -22.7204) -> (-16.7919, -23.1632)
  line L217 (-16.7919, -23.1632) -> (-18.4226, -25.6619)
  line L218 (-18.4226, -25.6619) -> (-16.0728, -27.1954)
  line L219 (-16.0728, -27.1954) -> (-14.4421, -24.6967)
  line L220 (-14.4421, -24.6967) -> (-13.7636, -25.1395)
  line L221 (-13.7636, -25.1395) -> (-17.0952, -30.2445)
  line L222 (-17.0952, -30.2445) -> (-17.7737, -29.8017)
  line L223 (-17.7737, -29.8017) -> (-16.4669, -27.7994)
  line L224 (-16.4669, -27.7994) -> (-18.8168, -26.2659)
  line L225 (-18.8168, -26.2659) -> (-20.1235, -28.2682)
  line L226 (-20.1235, -28.2682) -> (-20.802, -27.8254)
  line L227 (-20.802, -27.8254) -> (-17.4703, -22.7204)
  spline S212 degree 2 poles (-19.3142, -20.9453) (-18.8451, -21.3618) (-18.7923, -22.3665) (-19.3072, -22.9465) knots 0 0 0 1 2 2 2
  line L228 (-19.3072, -22.9465) -> (-20.9897, -24.8417)
  line L229 (-20.9897, -24.8417) -> (-20.6018, -25.1861)
  line L230 (-20.6018, -25.1861) -> (-21.0248, -25.6626)
  line L231 (-21.0248, -25.6626) -> (-21.4127, -25.3183)
  line L232 (-21.4127, -25.3183) -> (-22.2851, -26.3009)
  line L233 (-22.2851, -26.3009) -> (-22.8614, -25.7893)
  line L234 (-22.8614, -25.7893) -> (-21.9891, -24.8066)
  line L235 (-21.9891, -24.8066) -> (-23.0493, -23.8654)
  line L236 (-23.0493, -23.8654) -> (-22.6263, -23.3888)
  line L237 (-22.6263, -23.3888) -> (-21.566, -24.3301)
  line L238 (-21.566, -24.3301) -> (-20.1197, -22.7009)
  spline S213 degree 2 poles (-20.1197, -22.7009) (-19.8901, -22.4423) (-19.656, -22.1414) (-19.6106, -21.9637) knots 0 0 0 1 2 2 2
  spline S214 degree 2 poles (-19.6106, -21.9637) (-19.5672, -21.8107) (-19.7049, -21.4969) (-19.9044, -21.3198) knots 0 0 0 1 2 2 2
  spline S215 degree 2 poles (-19.9044, -21.3198) (-20.0447, -21.1952) (-20.3825, -21.0473) (-20.4645, -21.0207) knots 0 0 0 1 2 2 2
  line L239 (-20.4645, -21.0207) -> (-20.4978, -20.9912)
  line L240 (-20.4978, -20.9912) -> (-20.0386, -20.474)
  spline S216 degree 2 poles (-20.0386, -20.474) (-19.8367, -20.574) (-19.4583, -20.8174) (-19.3142, -20.9453) knots 0 0 0 1 2 2 2
  line L241 (-21.3573, -18.9904) -> (-20.695, -19.7101)
  line L242 (-20.695, -19.7101) -> (-21.5528, -20.4996)
  line L243 (-21.5528, -20.4996) -> (-22.2152, -19.7799)
  line L244 (-22.2152, -19.7799) -> (-21.3573, -18.9904)
  line L245 (-23.8655, -21.2986) -> (-23.2031, -22.0183)
  line L246 (-23.2031, -22.0183) -> (-24.061, -22.8078)
  line L247 (-24.061, -22.8078) -> (-24.7233, -22.0881)
  line L248 (-24.7233, -22.0881) -> (-23.8655, -21.2986)
  spline S217 degree 2 poles (-29.4771, -17.1312) (-29.3665, -17.324) (-29.0535, -17.6513) (-28.875, -17.7938) knots 0 0 0 1 2 2 2
  spline S218 degree 2 poles (-28.875, -17.7938) (-28.7038, -17.9235) (-28.4045, -18.0878) (-28.2794, -18.1471) knots 0 0 0 1 2 2 2
  line L249 (-28.2794, -18.1471) -> (-28.2549, -18.1899)
  line L250 (-28.2549, -18.1899) -> (-29.0048, -18.62)
  spline S219 degree 2 poles (-29.0048, -18.62) (-29.2618, -18.4598) (-29.9178, -17.7825) (-30.1218, -17.4269) knots 0 0 0 1 2 2 2
  spline S220 degree 2 poles (-30.1218, -17.4269) (-30.3282, -17.0669) (-30.4897, -16.4476) (-30.4608, -16.1406) knots 0 0 0 1 2 2 2
  spline S221 degree 2 poles (-30.4608, -16.1406) (-30.4263, -15.8134) (-30.0797, -15.2957) (-29.754, -15.1089) knots 0 0 0 1 2 2 2
  spline S222 degree 2 poles (-29.754, -15.1089) (-29.3169, -14.8583) (-28.3276, -15.0541) (-28.0109, -15.4078) knots 0 0 0 1 2 2 2
  line L251 (-28.0109, -15.4078) -> (-27.9595, -15.3783)
  spline S223 degree 2 poles (-27.9595, -15.3783) (-28.0211, -15.1915) (-28.0855, -14.7216) (-28.0246, -14.4703) knots 0 0 0 1 2 2 2
  spline S224 degree 2 poles (-28.0246, -14.4703) (-27.968, -14.2214) (-27.606, -13.7405) (-27.2589, -13.5414) knots 0 0 0 1 2 2 2
  spline S225 degree 2 poles (-27.2589, -13.5414) (-26.9032, -13.3375) (-26.1589, -13.2352) (-25.7997, -13.3254) knots 0 0 0 1 2 2 2
  spline S226 degree 2 poles (-25.7997, -13.3254) (-25.427, -13.4192) (-24.8024, -13.9323) (-24.5641, -14.348) knots 0 0 0 1 2 2 2
  spline S227 degree 2 poles (-24.5641, -14.348) (-24.3355, -14.7466) (-24.0811, -15.6371) (-24.0616, -15.979) knots 0 0 0 1 2 2 2
  line L252 (-24.0616, -15.979) -> (-24.8115, -16.409)
  line L253 (-24.8115, -16.409) -> (-24.841, -16.3576)
  spline S228 degree 2 poles (-24.841, -16.3576) (-24.806, -16.0414) (-24.9385, -15.1151) (-25.1523, -14.7423) knots 0 0 0 1 2 2 2
  spline S229 degree 2 poles (-25.1523, -14.7423) (-25.2776, -14.5237) (-25.6654, -14.1652) (-25.9075, -14.1105) knots 0 0 0 1 2 2 2
  spline S230 degree 2 poles (-25.9075, -14.1105) (-26.1472, -14.06) (-26.6103, -14.1262) (-26.8974, -14.2909) knots 0 0 0 1 2 2 2
  spline S231 degree 2 poles (-26.8974, -14.2909) (-27.1846, -14.4555) (-27.4616, -14.8365) (-27.4827, -15.0479) knots 0 0 0 1 2 2 2
  spline S232 degree 2 poles (-27.4827, -15.0479) (-27.5038, -15.2593) (-27.3518, -15.7131) (-27.2142, -15.9531) knots 0 0 0 1 2 2 2
  line L254 (-27.2142, -15.9531) -> (-27.0421, -16.2531)
  line L255 (-27.0421, -16.2531) -> (-27.6292, -16.5898)
  line L256 (-27.6292, -16.5898) -> (-27.7644, -16.3541)
  spline S233 degree 2 poles (-27.7644, -16.3541) (-28.0372, -15.8784) (-28.8355, -15.5389) (-29.2683, -15.7871) knots 0 0 0 1 2 2 2
  spline S234 degree 2 poles (-29.2683, -15.7871) (-29.4697, -15.9026) (-29.6684, -16.2215) (-29.6828, -16.395) knots 0 0 0 1 2 2 2
  spline S235 degree 2 poles (-29.6828, -16.395) (-29.6966, -16.5794) (-29.5827, -16.9469) (-29.4771, -17.1312) knots 0 0 0 1 2 2 2
  line L257 (-26.5462, -10.5859) -> (-26.1686, -11.4882)
  line L258 (-26.1686, -11.4882) -> (-27.2441, -11.9383)
  line L259 (-27.2441, -11.9383) -> (-27.6217, -11.036)
  line L260 (-27.6217, -11.036) -> (-26.5462, -10.5859)
  spline S236 degree 2 poles (-30.9839, -6.6198) (-29.4041, -6.179) (-27.6681, -6.6844) (-27.4012, -7.6408) knots 0 0 0 1 2 2 2
  spline S237 degree 2 poles (-27.4012, -7.6408) (-27.1303, -8.6115) (-28.3851, -9.9412) (-29.9315, -10.3727) knots 0 0 0 1 2 2 2
  spline S238 degree 2 poles (-29.9315, -10.3727) (-31.5208, -10.8162) (-33.2474, -10.3081) (-33.5156, -9.3469) knots 0 0 0 1 2 2 2
  spline S239 degree 2 poles (-33.5156, -9.3469) (-33.7851, -8.381) (-32.516, -7.0473) (-30.9839, -6.6198) knots 0 0 0 1 2 2 2
  spline S240 degree 2 poles (-28.9133, -7.1293) (-29.2354, -7.0961) (-30.1565, -7.2505) (-30.7608, -7.4192) knots 0 0 0 1 2 2 2
  spline S241 degree 2 poles (-30.7608, -7.4192) (-31.3651, -7.5878) (-32.2284, -7.9312) (-32.4949, -8.1338) knots 0 0 0 1 2 2 2
  spline S242 degree 2 poles (-32.4949, -8.1338) (-32.7615, -8.3364) (-32.9553, -8.8367) (-32.8637, -9.165) knots 0 0 0 1 2 2 2
  spline S243 degree 2 poles (-32.8637, -9.165) (-32.7721, -9.4933) (-32.3446, -9.8305) (-32.0008, -9.8679) knots 0 0 0 1 2 2 2
  spline S244 degree 2 poles (-32.0008, -9.8679) (-31.6678, -9.9033) (-30.7303, -9.734) (-30.1546, -9.5733) knots 0 0 0 1 2 2 2
  spline S245 degree 2 poles (-30.1546, -9.5733) (-29.536, -9.4007) (-28.7293, -9.0936) (-28.4403, -8.8796) knots 0 0 0 1 2 2 2
  spline S246 degree 2 poles (-28.4403, -8.8796) (-28.1676, -8.6804) (-27.9575, -8.1653) (-28.0531, -7.8227) knots 0 0 0 1 2 2 2
  spline S247 degree 2 poles (-28.0531, -7.8227) (-28.1434, -7.4991) (-28.5708, -7.1619) (-28.9133, -7.1293) knots 0 0 0 1 2 2 2
  line L261 (-34.589, -4.9698) -> (-32.2152, -4.8305)
  line L262 (-32.2152, -4.8305) -> (-32.1436, -5.3642)
  line L263 (-32.1436, -5.3642) -> (-34.47, -5.856)
  line L264 (-34.47, -5.856) -> (-34.589, -4.9698)
  line L265 (-34.7941, -3.4422) -> (-32.4203, -3.303)
  line L266 (-32.4203, -3.303) -> (-32.3486, -3.8366)
  line L267 (-32.3486, -3.8366) -> (-34.6751, -4.3284)
  line L268 (-34.6751, -4.3284) -> (-34.7941, -3.4422)
  dimension "d145" = 57.15
  constraints: 1 centre point, 1 coincident, 1 other
  measures "d145" diameter of A0
extrude "Extrusion19" cut sketch "Sketch26" against normal blind 1.27
split "Split1" plane through (0, 38.1, 0) removes the side toward (0, -1, 0)
equation "\"d85\" = spoolExteriorRadius"
equation "\"d86\" = spoolOverallHeight"
equation "\"d88\" = d85"
equation "\"d89\" = 0.5 * spoolOverallHeight"
equation "\"centerLineForSpool\" = 0.25 * spoolOverallHeight"
equation "\"d103\" = hexDiameter"
equation "\"d110\" = centerLineForSpool"
equation "\"d111\" = centerLineForSpool"
equation "\"d112\" = holeForString"
equation "\"d121\" = centerLineForSpool"
equation "\"d122\" = holeForString"
equation "\"d125\" = knotHoleDiameter"
equation "\"d127\" = holeForString"
equation "\"d128\" = centerLineForSpool"
equation "\"d129\" = knotHoleDiameter"
equation "\"d130\" = knotHoleDepth"
equation "\"d132\" = hexHoleChamfer"
equation "\"holeForString\" = stringDiameter + clearanceForString"
equation "\"stringDiameter\" = 3.048"
equation "\"clearanceForString\" = 2.032"
equation "\"spoolHeightWithoutSpacer\" = 69.85"
equation "\"hexShaftDiameter\" = 12.7"
equation "\"clearanceForHexShaft\" = 0.5715"
equation "\"hexDiameter\" = hexShaftDiameter + clearanceForHexShaft"
equation "\"supportChannels\" = 3.81"
equation "\"spoolInteriorDiameter\" = 38.1"
equation "\"spoolInteriroRadius\" = 0.5 * spoolInteriorDiameter"
equation "\"spoolExteriorDiameter\" = 82.55"
equation "\"spoolExteriorRadius\" = 0.5 * spoolExteriorDiameter"
equation "\"spoolFiletRadius\" = 0.5 * supportChannels"
equation "\"holeCenter\" = 0.25 * spoolHeightWithoutSpacer - 0.75 * supportChannels"
equation "\"hexHoleChamfer\" = 1.5875"
equation "\"stringHoleCenterFromHexShaft\" = 0.5 * hexDiameter + 0.5 * holeForString"
equation "\"textCircleDiameter\" = 0.75 * spoolExteriorDiameter"
equation "\"textHeight\" = 6.096"
equation "\"textDepth\" = 1.27"
equation "\"stringHoleChamfer\" = 4.7625"
equation "\"spoolTotalHeight\" = 76.2"
equation "\"spaceHeight\" = spoolTotalHeight - spoolHeightWithoutSpacer"
equation "\"spacerDiameter\" = 24.13"
equation "\"spoolOverallHeight\" = 76.2"
equation "\"d114\" = -spoolInteriroRadius"
equation "\"knotHoleDiameter\" = 9.525"
equation "\"d126\" = spoolInteriroRadius"
equation "\"d141\" = -0.5 * spoolTotalHeight"
equation "\"knotHoleDepth\" = 11.1125"
body "Solid3"
